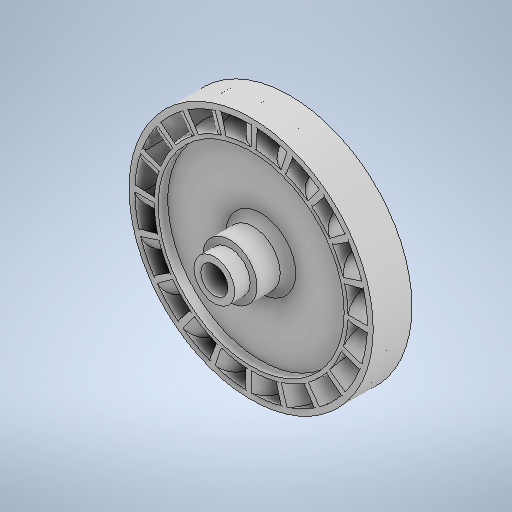
# Autodesk Inventor part: Turbine-V3
Saved by Autodesk Inventor 2026.1 (Build 301233020, 233B)
## iProperties
Created: 2025-10-12
Part Number: Turbine-V3
Material: Generic
Document SubType Name: Modeling
Designer: yo
Density: 1 g/cm^3
Appearance: Default
Author: yo
Autodesk Inventor part; units mm, degrees
ref_plane "YZ Plane" through (0, 0, 0) normal (1, 0, 0) x (0, 1, 0)
ref_plane "XZ Plane" through (0, 0, 0) normal (0, 1, 0) x (-1, 0, 0)
ref_plane "XY Plane" through (0, 0, 0) normal (0, 0, 1) x (1, 0, 0)
sketch "Sketch1" plane through (0, 0, 0) normal (0, 0, 1) x (1, 0, 0)
  circle A0 centre (0, 0) radius 3.5
  circle A1 centre (0, 0) radius 5
  circle A2 centre (0, 0) radius 25
  circle A3 centre (0, 0) radius 24
  circle A4 centre (0, 0) radius 30
  circle A5 centre (0, 0) radius 31.5
  dimension "d0" = 7
  dimension "d1" = 10
  dimension "d2" = 50
  dimension "d3" = 48
  dimension "d4" = 60
  dimension "d5" = 63
  constraints: 6 centre point, 6 coincident
  measures "d0" diameter of A0
  measures "d1" diameter of A1
  measures "d2" diameter of A2
  measures "d3" diameter of A3
  measures "d4" diameter of A4
  measures "d5" diameter of A5
extrude "Extrusion1" add sketch "Sketch1" along normal mid plane 5 contours A3
extrude "Extrusion2" add sketch "Sketch1" along normal mid plane 10 contours A4
sketch "Sketch2" plane through (0, 0, 5) normal (0, 0, 1) x (1, 0, 0)
  circle A0 centre (0, 0) radius 30 projected
  circle A1 centre (0, 0) radius 25 projected
  line L0 (25, 0) -> (30, 0)
  line L1 (24.1481, 6.4705) -> (28.9778, 7.7646)
  dimension "d10" = 15
  constraints: 4 end point, 4 line through centre, 4 point on circle, 1 horizontal
  measures "d10" angle of L0 L1
sketch "Sketch3" plane through (0, 0, 0) normal (1, 0, 0) x (0, 1, 0)
  line L0 (25, -5) -> (-25, -5) projected
  line L1 (-25, 5) -> (25, 5) projected
  arc A0 (0, -5) -> (0, 5) centre (-1, 0) ccw
  point P0 (0, 0)
  dimension "d11" = 1
  constraints: 3 midpoint, 3 vertical alignment, 2 point on circle, 1 centre point
  measures "d11" distance of A0.centre point (0, 0)
sweep "Sweep1" cut profiles "Sketch2" path "Sketch3" keep normal constant yes picked at (27.7141, 5.7718) path curves A0 contours L0 A1 L1 A0
extrude "Extrusion3" add sketch "Sketch1" along normal mid plane 10 contours A2 | A5
pattern_circular "Circular Pattern1" count 20 over 360 about axis through (0, 0, -10) along (0, 0, 1) of "Sweep1"
extrude "Extrusion4" add sketch "Sketch1" against normal blind 7 contours A1
extrude "Extrusion5" add sketch "Sketch1" along normal blind 2.5 contours A1
fillet "Fillet1" radius 3 2 edges at (-5, 0, -2.5) (-5, 0, -7)
sketch "Sketch4" plane through (0, 0, 2.5) normal (0, 0, 1) x (1, 0, 0)
  circle A0 centre (0, 0) radius 3.5 projected
  circle A1 centre (0, 0) radius 7
  dimension "d24" = 14
  constraints: 1 centre point, 1 coincident
  measures "d24" diameter of A1
extrude "Extrusion6" add sketch "Sketch4" along normal blind 12
sketch "Sketch5" plane through (0, 0, 14.5) normal (0, 0, 1) x (1, 0, 0)
  circle A0 centre (0, 0) radius 5.25
  circle A1 centre (0, 0) radius 7 projected
  dimension "d27" = 10.5
  constraints: 1 centre point, 1 coincident
  measures "d27" diameter of A0
extrude "Extrusion7" cut sketch "Sketch5" against normal blind 4
fillet "Fillet2" radius 2 1 edges at (-7, 0, 2.5)
body "Solid1"
